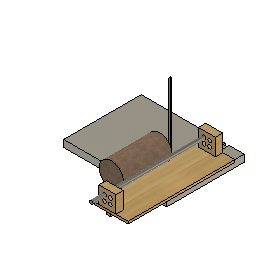
laguna14bx-log-jig (Autodesk Fusion 360 design; units mm, degrees)
Autodesk Fusion 360 part; units mm, degrees
note: some values were not read from the file. Set by a fixed rule: which sketch regions a step uses.
sketch "basicTable" plane through (0, 0, 0) normal (0, 0, 1) x (1, 0, 0) in component "table"
  line L0 (0, 0) -> (539.75, 0)
  line L1 (539.75, 0) -> (539.75, 406.4)
  line L2 (539.75, 406.4) -> (0, 406.4)
  line L3 (0, 406.4) -> (0, 0)
  dimension "d40" = 539.75
  dimension "d41" = 406.4
  constraint horizontal L0
  constraint vertical L1
  constraint horizontal L2
  constraint vertical L3
  constraint coincident L0.start L3.end
  measures "d40" distance of L0.start L0.end
  measures "d41" distance of L0.start L2.end
extrude "ExtrudeTableThickness" add sketch "basicTable" along normal blind 36.5125 makes body 1 in component "table"
sketch "miterOutline and Blade Placement" plane through (0, 0, 36.5125) normal (0, 0, 1) x (-1, 0, 0) in component "table"
  line L0 (0, -406.4) -> (0, 0)
  line L1 (0, 0) -> (-539.75, 0)
  line L2 (-539.75, 0) -> (-539.75, -406.4)
  line L3 (-539.75, -406.4) -> (0, -406.4)
  line L4 (-441.325, -406.4) -> (-460.375, -406.4)
  line L5 (-460.375, -406.4) -> (-460.375, 0)
  line L6 (-460.375, 0) -> (-441.325, 0)
  line L7 (-441.325, 0) -> (-441.325, -406.4)
  line L8 (-352.425, -406.4) -> (-352.425, 0) construction
  line L9 (-441.325, -203.2) -> (0, -203.2) construction
  point P0 (-352.425, -203.2)
  dimension "d44" = 79.375
  dimension "d45" = 19.05
  dimension "d46" = 88.9
  dimension "d47" = 203.2
  constraint horizontal L4
  constraint vertical L5
  constraint horizontal L6
  constraint vertical L7
  constraint coincident L1 L5.end
  constraint coincident L3 L4.start
  constraint coincident L3 L8.start
  constraint coincident L1 L8.end
  constraint perpendicular L1 L8
  constraint coincident L7 L9.start
  constraint coincident L0 L9.end
  constraint perpendicular L0 L9
  constraint midpoint L8 P0
  measures "d44" distance of L2 L5
  measures "d45" distance of L5 L7
  measures "d46" distance of L7 L8
  measures "d47" distance of L1 L9
extrude "ExtrudeMiterSlot" cut sketch "miterOutline and Blade Placement" against normal blind 12.7 contours L1 L3 L4 L5 L6 L7 bodies 1 in component "table"
sketch "Sketch1" plane through (0, 0, 36.5125) normal (0, 0, 1) x (-1, 0, 0) in component "miter"
  line L0 (-441.325, 0) -> (-441.325, -406.4)
  line L1 (-441.325, -406.4) -> (0, -406.4)
  line L2 (0, -406.4) -> (0, 0)
  line L3 (0, 0) -> (-441.325, 0)
  line L4 (-441.325, -406.4) -> (-460.375, -406.4)
  line L5 (-460.375, -406.4) -> (-460.375, 203.2)
  line L6 (-460.375, 203.2) -> (-441.325, 203.2)
  line L7 (-441.325, 203.2) -> (-441.325, -406.4)
  line L8 (-441.325, -101.6) -> (-460.375, -101.6) construction
  dimension "d50" = 19.05
  dimension "d81" = 609.6
  constraint horizontal L4
  constraint horizontal L6
  constraint vertical L7
  constraint coincident L0.end L1.start
  constraint midpoint L7 L8.start
  constraint midpoint L5 L8.end
  measures "d50" distance of L5 L7
  measures "d81" distance of L4.end L5.end
extrude "cut the miter" add sketch "Sketch1" against normal blind 12.7 separate body contours L0 L4 L5 L6 L7 makes body 2 in component "miter"
sketch "Sketch3" plane through (0, -203.2, 0) normal (0, -1, 0) x (1, 0, 0) in component "miter"
  line L0 (460.375, 36.5125) -> (441.325, 36.5125)
  line L1 (441.325, 36.5125) -> (441.325, 23.8125)
  line L2 (441.325, 23.8125) -> (460.375, 23.8125)
  line L3 (460.375, 23.8125) -> (460.375, 36.5125)
  line L4 (450.85, 36.5125, 0) -> (451.0909, 36.5125, -622.7895) construction
  line L5 (441.325, 23.8125, -609.6) -> (460.375, 23.8125, -609.6)
  line L6 (451.0909, 36.5125, -622.7895) -> (450.85, 23.8125, -609.6) construction
  line L7 (450.85, 23.8125, -609.6) -> (450.85, 23.8125, 0) construction
  line L8 (450.85, 36.5125) -> (450.85, 23.8125) construction
  constraint midpoint L0 L8.start
  constraint midpoint L2 L8.end
sketch "Sketch1 (2)" plane through (0, 0, 36.5125) normal (0, 0, 1) x (-1, 0, 0) in component "BandsawBlade"
  line L0 (-351.6312, -196.85) -> (-353.2187, -196.85)
  line L1 (-353.2187, -196.85) -> (-353.2187, -209.55)
  line L2 (-353.2187, -209.55) -> (-351.6312, -209.55)
  line L3 (-351.6312, -209.55) -> (-351.6312, -196.85)
  line L4 (-351.6312, -196.85) -> (-353.2187, -209.55) construction
  line L5 (-353.2187, -196.85) -> (-351.6312, -209.55) construction
  point P0 (-352.425, -203.2)
  point P1 (-352.425, -203.2)
  dimension "d76" = 1.5875
  dimension "d77" = 12.7
  constraint horizontal L0
  constraint perpendicular L0 L1
  constraint parallel L0 L2
  constraint parallel L1 L3
  constraint coincident L4 P1
  constraint coincident L5 P1
  constraint coincident P1 P0
  measures "d76" distance of L1.end L2.end
  measures "d77" distance of L0.end L1.end
extrude "Extrude1" add sketch "Sketch1 (2)" along normal blind 355.6 separate body makes body 3 in component "BandsawBlade"
sketch "sketch jig floor" plane through (0, 0, 36.5125) normal (0, 0, 1) x (-1, 0, 0) in component "floor"
  line L0 (-590.55, -406.4) -> (-352.425, -406.4)
  line L1 (-352.425, 152.4) -> (-590.55, 152.4)
  line L2 (-590.55, 152.4) -> (-590.55, -406.4)
  line L3 (-412.75, -457.2) -> (-590.55, -457.2)
  line L4 (-590.55, -457.2) -> (-590.55, 152.4)
  line L5 (-590.55, 152.4) -> (-412.75, 152.4)
  line L6 (-412.75, 152.4) -> (-412.75, -457.2)
  line L7 (-488.95, 152.4) -> (-488.95, -457.2) construction
  dimension "d188" = 177.8
  dimension "d189" = 609.6
  dimension "d191" = 76.2
  constraint horizontal L3
  constraint vertical L4
  constraint horizontal L5
  constraint vertical L6
  constraint coincident L1.end L2.start
  constraint coincident L5 L7.start
  constraint coincident L3 L7.end
  constraint perpendicular L3 L7
  measures "d188" distance of L3.start L3.end
  measures "d189" distance of L3.start L5.end
  measures "d191" distance of L6 L7
extrude "extrude floor" add sketch "sketch jig floor" along normal blind 12.7 separate body contours L0 L1 L2 L4 L5 L6 makes body 4 in component "floor"
sketch "Sketch1 (3)" plane through (0, -152.4, 0) normal (0, -1, 0) x (1, 0, 0) in component "frontFenceWall"
  line L0 (412.75, 36.5125) -> (590.55, 36.5125)
  line L1 (590.55, 49.2125) -> (412.75, 49.2125)
  line L2 (412.75, 49.2125) -> (412.75, 36.5125)
  line L3 (590.55, 49.2125) -> (501.65, 49.2125)
  line L4 (501.65, 49.2125) -> (501.65, 138.1125)
  line L5 (501.65, 138.1125) -> (590.55, 138.1125)
  line L6 (590.55, 138.1125) -> (590.55, 49.2125)
  line L7 (590.55, 36.5125) -> (590.55, 49.2125)
  dimension "d118" = 88.9
  dimension "d119" = 88.9
  constraint horizontal L3
  constraint vertical L4
  constraint horizontal L5
  constraint vertical L6
  constraint coincident L1.start L3.start
  measures "d118" distance of L1.start L3.end
  measures "d119" distance of L1.start L5.end
sketch "Sketch2" plane through (0, -152.4, 0) normal (0, -1, 0) x (1, 0, 0) in component "frontFenceWall"
  circle A0 centre (531.2833, 108.4792) radius 9.525
  line L0 (501.65, 49.2125) -> (501.65, 138.1125)
  line L1 (501.65, 138.1125) -> (590.55, 138.1125)
  dimension "d124" = 19.05
  dimension "d125" = 29.6333
  dimension "d129" = 29.6333
  measures "d124" diameter of A0
  measures "d125" distance of A0.centre L0
  measures "d129" distance of A0.centre L1
extrude "Extrude1'" add sketch "Sketch1 (3)" against normal blind 38.1 separate body contours L1 L3 L4 L5 L6 makes body 5 in component "frontFenceWall"
extrude "Extrude2" cut sketch "Sketch2" against normal blind 38.1 bodies 5 in component "frontFenceWall"
pattern_linear "R-Pattern1" count 2 spacing 29.6333 along (1, 0, 0) count 2 spacing 29.6333 along (0, 0, -1) of "Extrude2" in component "frontFenceWall"
sketch "Sketch4" plane through (0, 0, 0) normal (0, 0, 1) x (1, 0, 0) in component "frontFenceWall"
sketch "Sketch2 (2)" plane through (0, 0, 49.2125) normal (0, 0, 1) x (-1, 0, 0) in component "floor"
  line L0 (-412.75, 152.4) -> (-590.55, 152.4)
  line L1 (-590.55, -406.4) -> (-412.75, -406.4)
  line L2 (-412.75, -406.4) -> (-412.75, 152.4)
  line L3 (-175.1587, -111.0662) -> (-412.75, -127) construction
  line L4 (-590.55, 152.4) -> (-590.55, -406.4)
  constraint midpoint L2 L3.end
sketch "Sketch1 (4)" plane through (0, -152.4, 0) normal (0, -1, 0) x (1, 0, 0) in component "backFenceWall"
  line L0 (412.75, 36.5125) -> (590.55, 36.5125)
  line L1 (590.55, 49.2125) -> (412.75, 49.2125)
  line L2 (412.75, 49.2125) -> (412.75, 36.5125)
  line L3 (590.55, 49.2125) -> (501.65, 49.2125)
  line L4 (501.65, 49.2125) -> (501.65, 138.1125)
  line L5 (501.65, 138.1125) -> (590.55, 138.1125)
  line L6 (590.55, 138.1125) -> (590.55, 49.2125)
  line L7 (590.55, 36.5125) -> (590.55, 49.2125)
  dimension "d118_1" = 88.9
  dimension "d119_1" = 88.9
  constraint horizontal L3
  constraint vertical L4
  constraint horizontal L5
  constraint vertical L6
  constraint coincident L1.start L3.start
  measures "d118_1" distance of L1.start L3.end
  measures "d119_1" distance of L1.start L5.end
sketch "Sketch2 (3)" plane through (0, -152.4, 0) normal (0, -1, 0) x (1, 0, 0) in component "backFenceWall"
  circle A0 centre (531.2833, 108.4792) radius 9.525
  line L0 (501.65, 49.2125) -> (501.65, 138.1125)
  line L1 (501.65, 138.1125) -> (590.55, 138.1125)
  dimension "d124_1" = 19.05
  dimension "d125_1" = 29.6333
  dimension "d129_1" = 29.6333
  measures "d124_1" diameter of A0
  measures "d125_1" distance of A0.centre L0
  measures "d129_1" distance of A0.centre L1
extrude "Extrude1''" add sketch "Sketch1 (4)" against normal blind 38.1 separate body contours L1 L3 L4 L5 L6 makes body 6 in component "backFenceWall"
extrude "Extrude2'" cut sketch "Sketch2 (3)" against normal blind 19.05 bodies 6 in component "backFenceWall"
pattern_linear "R-Pattern1'" count 2 spacing 29.6333 along (1, 0, 0) count 2 spacing 29.6333 along (0, 0, -1) of "Extrude2'" in component "backFenceWall"
sketch "Sketch4 (2)" plane through (0, 0, 0) normal (0, 0, 1) x (1, 0, 0) in component "backFenceWall"
sketch "Sketch4 (3)" plane through (0, 0, 36.5125) normal (0, 0, 1) x (-1, 0, 0) in component "miter"
  line L0 (-441.325, -406.4) -> (-460.375, -406.4)
  line L1 (-450.85, 203.2) -> (-450.85, -406.4) construction
  point P0 (-450.85, 203.2)
  constraint coincident P0 L1.start
  constraint midpoint L0 L1.end
sketch "Sketch1 (5)" plane through (0, 0, 0) normal (0, 1, 0) x (1, 0, 0) in component "Log"
  circle A0 centre (169.0248, -100.0125) radius 63.5
  line L0 (0, -36.5125) -> (441.325, -36.5125)
  dimension "d204" = 127
  constraint tangent A0 L0
  measures "d204" diameter of A0
extrude "Extrude1'''" add sketch "Sketch1 (5)" along normal blind 254 separate body makes body 7 in component "Log"
sketch "LineForFencePosts" plane through (0, 0, 49.2125) normal (0, 0, 1) x (-1, 0, 0) in component "floor"
  line L0 (-412.75, 152.4) -> (-590.55, 152.4)
  line L1 (-590.55, -406.4) -> (-412.75, -406.4)
  line L2 (-438.15, 152.4) -> (-438.15, -406.4) construction
  line L3 (-412.75, 152.4) -> (-412.75, -457.2)
  dimension "d209" = 25.4
  constraint coincident L0 L2.start
  constraint coincident L1 L2.end
  constraint perpendicular L1 L2
  measures "d209" distance of L2 L3
sketch "Sketch1 (6)" plane through (0, 336.55, 0) normal (0, -1, 0) x (1, 0, 0) in component "pipe"
  circle A0 centre (429.6833, 108.4792) radius 9.525
  circle A1 centre (429.6833, 108.4792) radius 9.525
  dimension "d235" = 19.05
  constraint concentric A0 A1
  measures "d235" diameter of A1
extrude "Extrude1''''" add sketch "Sketch1 (6)" along normal blind 609.6 separate body makes body 8 in component "pipe"
component "table" placed x (1, 0, 0) y (0, 1, 0) z (0, 0, 1) at (0, 0, 0)
component "BandsawBlade" placed x (1, 0, 0) y (0, 1, 0) z (0, 0, 1) at (0, 0, 0)
component "floor" placed x (1, 0, 0) y (0, 1, 0) z (0, 0, 1) at (-38.1, -50.8, 0)
component "frontFenceWall" placed x (1, 0, 0) y (0, 1, 0) z (0, 0, 1) at (-101.6, -50.8, 0)
component "backFenceWall" placed x (1, 0, 0) y (0, 1, 0) z (0, 0, 1) at (-101.6, 469.9, 0)
component "Log" placed x (1, 0, 0) y (0, 1, 0) z (0, 0, 1) at (187.6335, -95.25, 8.4667)
component "pipe" placed x (1, 0, 0) y (0, 1, 0) z (0, 0, 1) at (0, 0, 0)
component "miter" placed x (1, 0, 0) y (0, 1, 0) z (0, 0, 1) at (38.1, 50.8, 0) in component "floor"
equation "tableWidth = 21.25 in"
equation "tableDepth = 16 in"
equation "miterWidth = 0.75 in"
equation "miterHeight = 0.5 in"
equation "tableHeight = 1 in + ( ( 7 / 16 ) * 1 in )"
equation "MiterEdgeToRightTableEdge = 3 in + ( ( 1 / 8 ) * 1 in )"
equation "MiterEdgeToBlade = 3.5 in"
equation "bladeDistanceFromFront = 8 in"
equation "d40 = tableWidth"
equation "d41 = tableDepth"
equation "d42 = tableHeight"
equation "d44 = MiterEdgeToRightTableEdge"
equation "d45 = miterWidth"
equation "d46 = MiterEdgeToBlade"
equation "d47 = bladeDistanceFromFront"
equation "d48 = -miterHeight"
equation "d50 = miterWidth"
equation "d51 = -miterHeight"
equation "subfloorThickness = 0.75 in"
equation "bladeThickness = ( 1 / 16 ) * 1 in"
equation "bladeWidth = ( 1 / 2 ) * 1 in"
equation "bladeHeight = 14 in"
equation "d76 = bladeThickness"
equation "d77 = bladeWidth"
equation "d78 = bladeHeight"
equation "jigDepth = 24 in"
equation "d81 = jigDepth"
equation "jigWidth = 7 in"
equation "maxResawOfBandsaw = 12 in"
equation "jigWallHeight = 3.5 in"
equation "halfInch = 0.5 in"
equation "d109 = halfInch"
equation "d118 = jigWallWidth"
equation "d119 = jigWallHeight"
equation "pipeClampDiameter = ( 3 / 4 ) * 1 in"
equation "d124 = pipeClampDiameter"
equation "d125 = jigWallWidth / ( pipeHoleColumns + 1 )"
equation "jigWallWidth = 3.5 in"
equation "pipeHoleColumns = 2"
equation "pipeHoleRows = 2"
equation "d129 = jigWallHeight / ( pipeHoleRows + 1 )"
equation "jigWallThickness = 1.5 in"
equation "d131 = -jigWallThickness"
equation "d133 = -jigWallThickness"
equation "d135 = pipeHoleColumns"
equation "d136 = pipeHoleRows"
equation "d137 = jigWallWidth / ( pipeHoleColumns + 1 )"
equation "d138 = jigWallHeight / ( pipeHoleRows + 1 )"
equation "d118_1 = jigWallWidth"
equation "d119_1 = jigWallHeight"
equation "d124_1 = pipeClampDiameter"
equation "d125_1 = jigWallWidth / ( pipeHoleColumns + 1 )"
equation "d129_1 = jigWallHeight / ( pipeHoleRows + 1 )"
equation "d131_1 = -jigWallThickness"
equation "d133_1 = -jigWallThickness / 2"
equation "d135_1 = pipeHoleColumns"
equation "d136_1 = pipeHoleRows"
equation "d137_1 = jigWallWidth / ( pipeHoleColumns + 1 )"
equation "d138_1 = jigWallHeight / ( pipeHoleRows + 1 )"
equation "d188 = jigWidth"
equation "d189 = jigDepth"
equation "MiterEdgeToLeftJigEdge = 3 in"
equation "d191 = MiterEdgeToLeftJigEdge"
equation "d204 = logDiameter"
equation "logDiameter = 5 in"
equation "logDepth = 10 in"
equation "d207 = logDepth"
equation "d209 = LeftJigWallToFenceEdge"
equation "LeftJigWallToFenceEdge = 1 in"
equation "d235 = pipeClampDiameter"
equation "d236 = pipeLength"
equation "pipeLength = 24 in"
equation "d243 = logDiameter / 2"
equation "d245 = logDepth / 2"
equation "d247 = -pipeClampDiameter / 2"
equation "d249 = -pipeLength / 2"
named bodies: "frontFenceWall"
